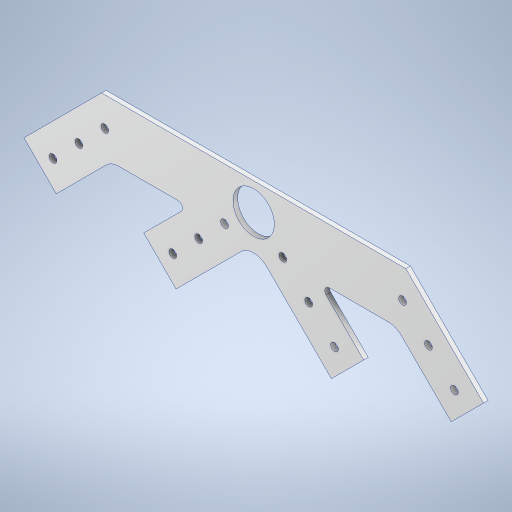
# Autodesk Inventor part: CH1-01-KneePivotPlate
Saved by Autodesk Inventor 2023 (Build 270158000, 158)
## iProperties
Created: 2023-03-03
Part Number: CH1-01-KneePivotPlate
Material: Aluminum 6061
Document SubType Name: Modeling
Designer: megan
Density: 2.7 g/cm^3
Appearance: Aluminum - Flat
Mass: 134.421 g
Surface Area: 352.442 cm^2
Volume: 49.7856 cm^3
Author: megan
Autodesk Inventor part; units mm, degrees
ref_plane "YZ Plane" through (0, 0, 0) normal (1, 0, 0) x (0, 1, 0)
ref_plane "XZ Plane" through (0, 0, 0) normal (0, 1, 0) x (-1, 0, 0)
ref_plane "XY Plane" through (0, 0, 0) normal (0, 0, 1) x (1, 0, 0)
sketch "Sketch1" plane through (0, 0, 0) normal (0, 0, 1) x (1, 0, 0)
  circle A0 centre (0, 0) radius 14.31
  line L0 (-76.3322, -50.4809) -> (-44.9013, -19.05)
  line L1 (0, -91.3278) -> (0, 37.4463) projected
  line L2 (0, -19.05) -> (-53.8815, -72.9315)
  line L3 (-53.8815, -72.9315) -> (-76.3322, -50.4809)
  line L4 (0, 19.05) -> (-105.5841, 19.05)
  line L5 (-105.5841, 19.05) -> (-159.4656, -34.8315)
  line L6 (-159.4656, -34.8315) -> (-137.015, -57.2822)
  line L7 (-137.015, -57.2822) -> (-98.7828, -19.05)
  line L8 (-98.7828, -19.05) -> (-44.9013, -19.05)
  line L9 (76.3322, -50.4809) -> (44.9013, -19.05)
  line L10 (0, -19.05) -> (53.8815, -72.9315)
  line L11 (53.8815, -72.9315) -> (76.3322, -50.4809)
  line L12 (0, 19.05) -> (105.5841, 19.05)
  line L13 (105.5841, 19.05) -> (159.4656, -34.8315)
  line L14 (159.4656, -34.8315) -> (137.015, -57.2822)
  line L15 (137.015, -57.2822) -> (98.7828, -19.05)
  line L16 (98.7828, -19.05) -> (44.9013, -19.05)
  line L17 (0, -19.05) -> (-10.6721, -29.7221)
  point P0 (-66.8959, -41.0446)
  dimension "d1" = 28.62
  dimension "d4" = 76.2
  dimension "d6" = 45
  dimension "d15" = 31.75
  dimension "d59" = 31.75
  dimension "d61" = 101.6
  dimension "d62" = 38.1
  dimension "d63" = 19.05
  dimension "d83" = 19.05
  constraints: 34 end point, 7 symmetric about line, 4 parallel, 4 point on line, 3 perpendicular, 1 centre point, 1 horizontal
  measures "d1" diameter of A0
  measures "d4" distance of L2.start L2.end
  measures "d6" angle of L2 L1
  measures "d15" distance between parallel lines of L2 L0
  measures "d59" distance of L5.end L6.end
  measures "d61" distance between parallel lines of L2 L5
  measures "d62" distance between parallel lines of L8 L4
  measures "d63" distance of point (0, 0) L2.start
  measures "d83" distance from line of L16 point (0, 0)
extrude "Extrusion1" add sketch "Sketch1" along normal blind 3.175 contours A0 L1 L12 L13 L14 L15 L16 L9 L11 L10 | A0 L1 L2 L3 L0 L8 L7 L6 L5 L4
sketch "Sketch3" plane through (0, 0, 3.175) normal (0, 0, 1) x (1, 0, 0)
  line L0 (53.8815, -72.9315) -> (76.3322, -50.4809) projected
  line L1 (76.3322, -50.4809) -> (44.9013, -19.05) projected
  line L2 (44.9013, -19.05) -> (98.7828, -19.05) projected
  line L3 (98.7828, -19.05) -> (137.015, -57.2822) projected
  line L4 (137.015, -57.2822) -> (159.4656, -34.8315) projected
  line L5 (159.4656, -34.8315) -> (105.5841, 19.05) projected
  line L6 (105.5841, 19.05) -> (-105.5841, 19.05) projected
  line L7 (-105.5841, 19.05) -> (-159.4656, -34.8315) projected
  line L8 (-159.4656, -34.8315) -> (-137.015, -57.2822) projected
  line L9 (-137.015, -57.2822) -> (-98.7828, -19.05) projected
  line L10 (-98.7828, -19.05) -> (-44.9013, -19.05) projected
  line L11 (-44.9013, -19.05) -> (-76.3322, -50.4809) projected
  line L12 (-76.3322, -50.4809) -> (-53.8815, -72.9315) projected
  line L13 (-53.8815, -72.9315) -> (0, -19.05) projected
  line L14 (0, -19.05) -> (53.8815, -72.9315) projected
  circle A0 centre (0, 0) radius 14.31 projected
  line L15 (-148.2403, -46.0569) -> (-83.1335, 19.05)
  line L16 (-65.1069, -61.7062) -> (15.6494, 19.05)
  circle A1 centre (-139.2601, -37.0766) radius 2.65
  circle A2 centre (-121.2995, -19.1161) radius 2.65
  circle A3 centre (-103.339, -1.1556) radius 2.65
  circle A4 centre (-56.1266, -52.726) radius 2.65
  circle A5 centre (-38.1661, -34.7654) radius 2.65
  circle A6 centre (-20.2056, -16.8049) radius 2.65
  dimension "d64" = 5.3
  dimension "d67" = 25.4
  dimension "d72" = 12.7
  dimension "d73" = 12.7
  dimension "d76" = 25.4
  constraints: 6 centre point, 4 end point, 4 point on line, 2 midpoint, 2 parallel, 1 equal radius, 10 other
  measures "d64" diameter of A1
  measures "d67" distance of A1.centre A2.centre
  measures "d72" distance from line of L8 A1.centre
  measures "d73" distance from line of L12 A4.centre
  measures "d76" distance of A4.centre A5.centre
extrude "Extrusion3" cut sketch "Sketch3" against normal blind 25.4 contours A4 L16 | L16 A4 | A5 L16 | L16 A5 | A6 L16 | L16 A6 | A3 L15 | L15 A3 | A1 L15 | L15 A1 | A2 L15 | L15 A2
mirror "Mirror2" about plane through (0, 0, 0) normal (1, 0, 0) of "Extrusion3"
fillet "Fillet1" radius 12.7 3 edges at (-98.7828, -19.05, 1.5875) (0, -19.05, 1.5875) (98.7828, -19.05, 1.5875)
fillet "Fillet2" radius 3.175 2 edges at (-44.9013, -19.05, 1.5875) (44.9013, -19.05, 1.5875)
equation "\"d1\" = bearingDiameter"
equation "\"d4\" = boltedLength"
equation "\"d6\" = 0.5 * theta12"
equation "\"d59\" = d15"
equation "\"d61\" = gearboxLength"
equation "\"d63\" = 0.5 * d62"
equation "\"d83\" = d63"
equation "\"topDiameter\" = 45"
equation "\"bearingDiameter\" = 28.62"
equation "\"plateThickness\" = 6.35"
equation "\"theta12\" = 90deg"
equation "\"gearboxLength\" = 101.6"
equation "\"boltedLength\" = 76.2"
equation "\"topDiameter_1\" = 25"
equation "\"shaftLength_1\" = 76.2"
equation "\"bearingDiameter_1\" = 28.62"
equation "\"plateThickness_1\" = 6.35"
equation "\"theta12_1\" = 100deg"
equation "\"boltDiameter_1\" = 6"
equation "\"gearboxLength_1\" = 101.6"
equation "\"boltedLength_1\" = 76.2"
equation "\"innerBoltSpacing_1\" = 12.7"
equation "\"outerBoltSpacing_1\" = 12.7"
equation "\"shaftLength\" = 76.2"
equation "\"boltDiameter\" = 5.3"
equation "\"outerBoltSpacing\" = 12.7"
equation "\"innerBoltSpacing\" = 12.7"
body "Solid1"
